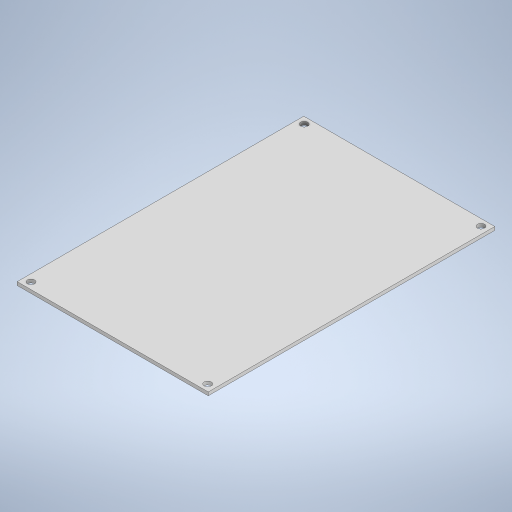
# Autodesk Inventor part: board
Saved by Autodesk Inventor 2023 (Build 270158000, 158)
## iProperties
Created: 2026-02-13
Part Number: board
Material: Типовые
Document SubType Name: Modeling
Designer: garin
Density: 1 g/cm^3
Appearance: По умолчанию
Author: garin
Autodesk Inventor part; units mm, degrees
ref_plane "YZ Plane" through (0, 0, 0) normal (1, 0, 0) x (0, 1, 0)
ref_plane "XZ Plane" through (0, 0, 0) normal (0, 1, 0) x (-1, 0, 0)
ref_plane "XY Plane" through (0, 0, 0) normal (0, 0, 1) x (1, 0, 0)
sketch "Эскиз1" plane through (0, 0, 0) normal (0, 1, 0) x (-1, 0, 0)
  line L0 (40, 60) -> (-40, 60)
  line L1 (-40, 60) -> (-40, -60)
  line L2 (-40, -60) -> (40, -60)
  line L3 (40, -60) -> (40, 60)
  line L4 (40, 0) -> (-40, 0) construction
  line L5 (0, 60) -> (0, -60) construction
  line L6 (40, 60) -> (37, 60) construction
  line L7 (40, 57) -> (40, 60) construction
  line L8 (40, 57.2) -> (40, -57.2) construction
  line L9 (40, 57.2) -> (37, 57.2) construction
  line L10 (53.0108, 0) -> (-51.4211, 0) construction
  line L11 (0, 75.3186) -> (0, -88.6188) construction
  circle A0 centre (37, 57.2) radius 1.5
  circle A1 centre (37, -57.2) radius 1.5
  circle A2 centre (-37, 57.2) radius 1.5
  circle A3 centre (-37, -57.2) radius 1.5
  point P0 (0, 0)
  point P1 (0, 0)
  point P2 (56.9303, -23.4668)
  dimension "d0" = 80
  dimension "d1" = 120
  dimension "d5" = 3
  dimension "d6" = 3
  constraints: 24 end point, 5 midpoint, 4 centre point, 3 coincident, 3 horizontal, 3 symmetric about line, 2 parallel, 2 perpendicular, 2 vertical, 3 other
  measures "d0" distance of L2.end L1.end
  measures "d1" distance of L1.end L0.end
  measures "d5" distance of L8.start L9.end
  measures "d6" diameter of A0
extrude "Выдавливание1" add sketch "Эскиз1" along normal blind 1.4
